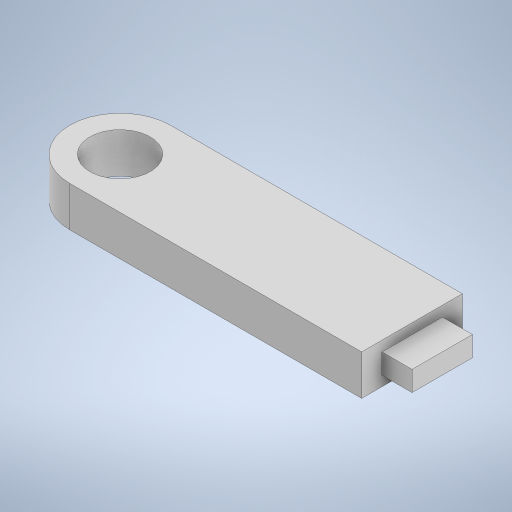
# Autodesk Inventor part: AlignmentGateClosedBeforeServo
Saved by Autodesk Inventor 2023 (Build 270158000, 158)
## iProperties
Created: 2023-05-02
Part Number: AlignmentGateClosedBeforeServo
Material: Generic
Document SubType Name: Modeling
Designer: 1roweste
Density: 1 g/cm^3
Appearance: Default
Author: 1roweste
Autodesk Inventor part; units mm, degrees
ref_plane "YZ Plane" through (0, 0, 0) normal (1, 0, 0) x (0, 1, 0)
ref_plane "XZ Plane" through (0, 0, 0) normal (0, 1, 0) x (-1, 0, 0)
ref_plane "XY Plane" through (0, 0, 0) normal (0, 0, 1) x (1, 0, 0)
sketch "Sketch1" plane through (0, 0, 0) normal (0, 1, 0) x (-1, 0, 0)
  circle A0 centre (0, 0) radius 1.5
  circle A1 centre (0, 0) radius 2.5
  line L0 (0, 0) -> (2.5, 0)
  line L1 (0, 0.75) -> (2.5, 0.75)
  line L2 (0, -0.75) -> (2.5, -0.75)
  line L3 (0, 2.5) -> (-14.5, 2.5)
  line L4 (-14.5, 2.5) -> (-14.5, -2.5)
  line L5 (-14.5, -2.5) -> (0, -2.5)
  line L6 (0, -2.5) -> (0, 2.5)
  point P0 (1.299, 0.75)
  point P1 (2.3848, 0.75)
  point P2 (2.3848, -0.75)
  point P3 (1.299, -0.75)
  dimension "d0" = 3
  dimension "d1" = 5
  dimension "d2" = 0.75
  dimension "d3" = 0.75
  dimension "d13" = 14.5
  constraints: 14 end point, 4 parallel, 2 centre point, 2 coincident, 2 horizontal, 2 point on circle, 1 perpendicular
  measures "d0" diameter of A0
  measures "d1" diameter of A1
  measures "d2" distance between parallel lines of L0 L1
  measures "d3" distance between parallel lines of L0 L2
  measures "d13" distance from line of L4 L0.start
extrude "Extrusion1" add sketch "Sketch1" along normal blind 2 contours L0 A1 L2 A0 | A0 L1 A1 L0 | A0 L6 A1 L1 | L2 A1 L6 A0 | A0 L6 A1 | A1 L5 L4 L3
sketch "Sketch2" plane through (14.5, 0, 2.5) normal (1, 0, 0) x (0, 0, -1)
  line L0 (1, 1.5) -> (4, 1.5)
  line L1 (4, 1.5) -> (4, 0.5)
  line L2 (4, 0.5) -> (1, 0.5)
  line L3 (1, 0.5) -> (1, 1.5)
  line L4 (0, 0) -> (5, 0) projected
  line L5 (5, 0) -> (5, 2) projected
  point P0 (2.5, 0)
  dimension "d6" = 3
  dimension "d7" = 1
  dimension "d8" = 0.5
  dimension "d9" = 1
  constraints: 8 end point, 2 parallel, 1 horizontal, 1 perpendicular
  measures "d6" distance of L1.end L2.end
  measures "d7" distance of L0.end L1.end
  measures "d8" distance between parallel lines of L4 L2
  measures "d9" distance between parallel lines of L5 L1
extrude "Extrusion2" add sketch "Sketch2" along normal blind 1.5
body "Solid1"
